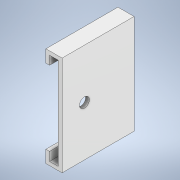
# Autodesk Inventor part: servo_mount
Saved by Autodesk Inventor 2021 (Build 250183000, 183)
## iProperties
Created: 2024-06-13
Part Number: servo_mount
Material: PC/ABS Plastic
Document SubType Name: Modeling
Designer: ASUS
Density: 0.357273 g/cm^3
Appearance: Smooth - White
Author: ASUS
Autodesk Inventor part; units mm, degrees
ref_plane "YZ Plane" through (0, 0, 0) normal (1, 0, 0) x (0, 1, 0)
ref_plane "XZ Plane" through (0, 0, 0) normal (0, 1, 0) x (-1, 0, 0)
ref_plane "XY Plane" through (0, 0, 0) normal (0, 0, 1) x (1, 0, 0)
sketch "Sketch1" plane through (0, 0, 0) normal (0, 0, 1) x (1, 0, 0)
  line L0 (0, 0) -> (13, 0)
  line L1 (13, 0) -> (13, 80)
  line L2 (13, 80) -> (0, 80)
  line L3 (0, 80) -> (0, 0)
  dimension "d0" = 80
  dimension "d1" = 13
  constraints: 8 end point, 2 parallel, 1 horizontal, 1 perpendicular
  measures "d0" distance between parallel lines of L0 L2
  measures "d1" distance between parallel lines of L3 L1
extrude "Extrusion1" add sketch "Sketch1" along normal blind 58
sketch "Sketch2" plane through (0, 0, 58) normal (0, 0, 1) x (1, 0, 0)
  line L0 (10, 77) -> (3, 77)
  line L1 (3, 3) -> (10, 3)
  line L2 (10, 3) -> (10, 77)
  line L3 (13, 0) -> (13, 80) projected
  line L4 (13, 80) -> (0, 80) projected
  line L5 (0, 0) -> (13, 0) projected
  line L6 (0, 80) -> (0, 0) projected
  line L7 (0, 10) -> (3, 10)
  line L8 (3, 70) -> (0, 70)
  line L9 (0, 70) -> (0, 10)
  line L10 (3, 77) -> (3, 70)
  line L11 (3, 10) -> (3, 3)
  point P0 (0, 70)
  dimension "d4" = 3
  dimension "d5" = 3
  dimension "d6" = 3
  dimension "d8" = 10
  dimension "d9" = 10
  constraints: 16 end point, 4 parallel, 2 horizontal, 2 perpendicular, 1 point on line
  measures "d4" distance between parallel lines of L3 L2
  measures "d5" distance between parallel lines of L4 L0
  measures "d6" distance between parallel lines of L5 L1
  measures "d8" distance between parallel lines of L4 L8
  measures "d9" distance between parallel lines of L5 L7
extrude "Extrusion2" cut sketch "Sketch2" against normal through all contours L2 L1 L11 L7 L6 L8 L10 L0
sketch "Sketch3" plane through (13, 0, 0) normal (1, 0, 0) x (0, 0, -1)
  circle A0 centre (-40, 40) radius 4
  line L0 (-58, 0) -> (-58, 80) projected
  line L1 (0, 0) -> (-58, 0) projected
  line L2 (0, 0) -> (0, 80) projected
  dimension "d12" = 8
  dimension "d14" = 40
  dimension "d17" = 40
  constraints: 1 centre point
  measures "d12" diameter of A0
  measures "d14" distance from line of L1 A0.centre
  measures "d17" distance from line of L2 A0.centre
extrude "Extrusion3" cut sketch "Sketch3" against normal through all
body "Solid1"
